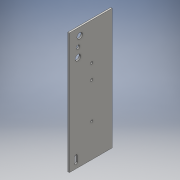
# Autodesk Inventor part: BackPanel
Saved by Autodesk Inventor 2016 (Build 200138000, 138)
## iProperties
Created: 2017-04-08
Part Number: BackPanel
Material: Generic
Document SubType Name: Modeling
Designer: Thoma
Density: 1 g/cm^3
Appearance: Default
Author: Thoma
Autodesk Inventor part; units mm, degrees
ref_plane "YZ Plane" through (0, 0, 0) normal (1, 0, 0) x (0, 1, 0)
ref_plane "XZ Plane" through (0, 0, 0) normal (0, 1, 0) x (-1, 0, 0)
ref_plane "XY Plane" through (0, 0, 0) normal (0, 0, 1) x (1, 0, 0)
sketch "Sketch1" plane through (0, 0, 0) normal (1, 0, 0) x (0, 1, 0)
  line L0 (0, 0) -> (45.3, 0)
  line L1 (45.3, 0) -> (45.3, -128)
  line L2 (45.3, -128) -> (0, -128)
  line L3 (0, -128) -> (0, 0)
  circle A0 centre (11, -8) radius 3
  circle A1 centre (9, -17.5) radius 2
  circle A2 centre (9, -27) radius 3
  circle A3 centre (23.5, -39.25) radius 1.25
  circle A4 centre (23.5, -54.75) radius 1.25
  circle A5 centre (23.5, -92.75) radius 1.25
  line L4 (5.5, -115) -> (8.5, -115) construction
  line L5 (8.5, -115) -> (8.5, -124) construction
  line L6 (8.5, -124) -> (5.5, -124) construction
  line L7 (5.5, -124) -> (5.5, -115) construction
  line L8 (5.5, -116.5) -> (5.5, -122.5)
  line L9 (8.5, -116.5) -> (8.5, -122.5)
  arc A6 (8.5, -116.5) -> (5.5, -116.5) centre (7, -116.5) ccw
  arc A7 (5.5, -122.5) -> (8.5, -122.5) centre (7, -122.5) ccw
  dimension "d0" = 45.3
  dimension "d1" = 128
  dimension "d2" = 6
  dimension "d3" = 4
  dimension "d4" = 6
  dimension "d5" = 8
  dimension "d6" = 17.5
  dimension "d7" = 27
  dimension "d8" = 11
  dimension "d9" = 9
  dimension "d10" = 9
  dimension "d11" = 2.5
  dimension "d12" = 39.25
  dimension "d13" = 23.5
  dimension "d14" = 2.5
  dimension "d15" = 54.75
  dimension "d16" = 23.5
  dimension "d17" = 2.5
  dimension "d18" = 23.5
  dimension "d19" = 92.75
  dimension "d20" = 3
  dimension "d21" = 9
  dimension "d22" = 115
  dimension "d23" = 5.5
  dimension "d27" = 6
  dimension "d28" = 1.5
  dimension "d29" = 6
  constraints: 20 end point, 8 centre point, 4 parallel, 4 point on circle, 4 point on line, 3 tangent, 2 horizontal, 2 perpendicular
  measures "d0" distance of L1.end L2.end
  measures "d1" distance of L0.end L1.end
  measures "d2" diameter of A0
  measures "d3" diameter of A1
  measures "d4" diameter of A2
  measures "d5" distance from line of L0 A0.centre
  measures "d6" distance from line of L0 A1.centre
  measures "d7" distance from line of L0 A2.centre
  measures "d8" distance from line of L3 A0.centre
  measures "d9" distance from line of L3 A1.centre
  measures "d10" distance from line of L3 A2.centre
  measures "d11" diameter of A3
  measures "d12" distance from line of A3.centre L0
  measures "d13" distance from line of L3 A3.centre
  measures "d14" diameter of A4
  measures "d15" distance from line of L0 A4.centre
  measures "d16" distance from line of L3 A4.centre
  measures "d17" diameter of A5
  measures "d18" distance from line of L3 A5.centre
  measures "d19" distance from line of L0 A5.centre
  measures "d20" distance of L5.end L6.end
  measures "d21" distance of L4.end L5.end
  measures "d22" distance between parallel lines of L4 L0
  measures "d23" distance between parallel lines of L3 L7
  measures "d27" distance of L8.start L8.end
  measures "d28" distance from line of L8.start L4
  measures "d29" distance of L9.start L9.end
extrude "Extrusion2" add sketch "Sketch1" along normal blind 1.6
body "Solid2"
